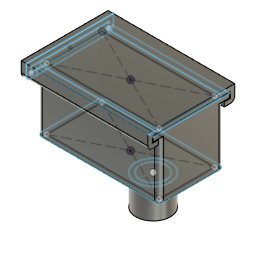
IRboxAugust v4 (Autodesk Fusion 360 design; units mm, degrees)
Autodesk Fusion 360 part; units mm, degrees
sketch "Sketch1" plane through (0, 0, 0) normal (0, 0, 1) x (1, 0, 0)
  line L0 (37.5, -18.5) -> (-37.5, -18.5)
  line L1 (-37.5, -18.5) -> (-37.5, 18.5)
  line L2 (-37.5, 18.5) -> (37.5, 18.5)
  line L3 (37.5, 18.5) -> (37.5, -18.5)
  line L4 (37.5, -18.5) -> (-37.5, 18.5) construction
  line L5 (-37.5, -18.5) -> (37.5, 18.5) construction
  line L6 (-37.5, 21.5) -> (37.5, 21.5)
  line L7 (40.5, 18.5) -> (40.5, -18.5)
  line L8 (37.5, -21.5) -> (-37.5, -21.5)
  line L9 (-40.5, -18.5) -> (-40.5, 18.5)
  arc A0 (-37.5, 21.5) -> (-40.5, 18.5) centre (-37.5, 18.5) ccw
  arc A1 (40.5, 18.5) -> (37.5, 21.5) centre (37.5, 18.5) ccw
  arc A2 (37.5, -21.5) -> (40.5, -18.5) centre (37.5, -18.5) ccw
  arc A3 (-40.5, -18.5) -> (-37.5, -21.5) centre (-37.5, -18.5) ccw
  circle A4 centre (20, -5) radius 8.5
  circle A5 centre (20, -5) radius 11.5
  dimension "d1" = 75
  dimension "d2" = 37
  dimension "d4" = 3
  dimension "d5" = 3
  dimension "d6" = 3
  dimension "d7" = 3
  dimension "d10" = 17
  dimension "d11" = 23
  constraint horizontal L0
  constraint perpendicular L0 L1
  constraint parallel L0 L2
  constraint parallel L1 L3
  constraint coincident L4 origin
  constraint coincident L5 origin
  constraint parallel L2 L6
  constraint parallel L3 L7
  constraint parallel L0 L8
  constraint parallel L1 L9
  constraint tangent L6 A0
  constraint tangent L9 A0
  constraint tangent L6 A1
  constraint tangent L7 A1
  constraint tangent L7 A2
  constraint tangent L8 A2
  constraint tangent L8 A3
  constraint tangent L9 A3
  constraint concentric A4 A5
  measures "d1" distance of L1.end L2.end
  measures "d2" distance of L0.end L1.end
  measures "d4" radius of A0
  measures "d5" radius of A1
  measures "d6" radius of A2
  measures "d7" radius of A3
  measures "d10" diameter of A4
  measures "d11" diameter of A5
extrude "Extrude2" add sketch "Sketch1" against normal blind 20 contours A5 makes body 1
extrude "Extrude1" add sketch "Sketch1" along normal blind 3 separate body contours L0 L1 L2 L3 | L6 L7 L8 L9 A0 A1 A2 A3 | A4 | A5 makes body 2
extrude "Extrude3" cut sketch "Sketch1" along normal blind 11 contours A4 bodies 2
extrude "Extrude4" add sketch "Sketch1" along normal blind 41 contours L6 L7 L8 L9 A0 A1 A2 A3 bodies 2
sketch "Sketch2" plane through (0, 0, 41) normal (0, 0, 1) x (-1, 0, 0)
  line L0 (37.5, -18.5) -> (-37.5, -18.5)
  line L1 (-37.5, -18.5) -> (-37.5, 18.5)
  line L2 (-37.5, 18.5) -> (37.5, 18.5)
  line L3 (37.5, 18.5) -> (37.5, -18.5)
  arc A0 (37.5, -21.5) -> (40.5, -18.5) centre (37.5, -18.5) ccw
  line L4 (40.5, -18.5) -> (40.5, 18.5)
  arc A1 (40.5, 18.5) -> (37.5, 21.5) centre (37.5, 18.5) ccw
  line L5 (37.5, 21.5) -> (-37.5, 21.5)
  arc A2 (-37.5, 21.5) -> (-40.5, 18.5) centre (-37.5, 18.5) ccw
  line L6 (-40.5, 18.5) -> (-40.5, -18.5)
  arc A3 (-40.5, -18.5) -> (-37.5, -21.5) centre (-37.5, -18.5) ccw
  line L7 (-37.5, -21.5) -> (37.5, -21.5)
  line L8 (37.5, -18.5) -> (-37.5, -18.5)
  line L9 (-37.5, -18.5) -> (-37.5, 18.5)
  line L10 (-37.5, 18.5) -> (37.5, 18.5)
  line L11 (37.5, 18.5) -> (37.5, -18.5)
  line L12 (37.5, -18.5) -> (-37.5, 18.5) construction
  line L13 (-37.5, -18.5) -> (37.5, 18.5) construction
  line L14 (37.5, -21.5) -> (-37.5, -21.5)
  line L15 (-40.5, -18.5) -> (-40.5, 18.5)
  line L16 (-37.5, 21.5) -> (37.5, 21.5)
  line L17 (40.5, 18.5) -> (40.5, -18.5)
  arc A4 (37.5, -21.5) -> (40.5, -18.5) centre (37.5, -18.5) ccw
  arc A5 (40.5, 18.5) -> (37.5, 21.5) centre (37.5, 18.5) ccw
  arc A6 (-40.5, -18.5) -> (-37.5, -21.5) centre (-37.5, -18.5) ccw
  arc A7 (-37.5, 21.5) -> (-40.5, 18.5) centre (-37.5, 18.5) ccw
  line L18 (37.5, -21.5) -> (-37.5, -21.5)
  line L19 (-37.5, -21.5) -> (-37.5, -25.5)
  line L20 (-37.5, -25.5) -> (37.5, -25.5)
  line L21 (37.5, -25.5) -> (37.5, -21.5)
  line L22 (37.5, 21.5) -> (-37.5, 21.5)
  line L23 (-37.5, 21.5) -> (-37.5, 25.5)
  line L24 (-37.5, 25.5) -> (37.5, 25.5)
  line L25 (37.5, 25.5) -> (37.5, 21.5)
  line L26 (-37.5, -25.5) -> (-40.5, -25.5)
  line L27 (-40.5, -25.5) -> (-40.5, 25.5)
  line L28 (-40.5, 25.5) -> (-37.5, 25.5)
  line L29 (-37.5, 25.5) -> (-37.5, -25.5)
  dimension "d19" = 3
  dimension "d20" = 3
  dimension "d21" = 3
  dimension "d22" = 3
  dimension "d23" = 4
  dimension "d24" = 4
  constraint horizontal L8
  constraint perpendicular L8 L9
  constraint parallel L8 L10
  constraint parallel L9 L11
  constraint coincident L0.start L3.end
  constraint coincident L12 origin
  constraint coincident L13 origin
  constraint parallel L8 L14
  constraint parallel L9 L15
  constraint parallel L10 L16
  constraint parallel L11 L17
  constraint tangent L14 A4
  constraint tangent L17 A4
  constraint tangent L16 A5
  constraint tangent L17 A5
  constraint tangent L14 A6
  constraint tangent L15 A6
  constraint tangent L15 A7
  constraint tangent L16 A7
  constraint horizontal L18
  constraint vertical L19
  constraint horizontal L20
  constraint vertical L21
  constraint horizontal L22
  constraint vertical L23
  constraint horizontal L24
  constraint vertical L25
  constraint horizontal L26
  constraint vertical L27
  constraint horizontal L28
  constraint vertical L29
  measures "d19" radius of A4
  measures "d20" radius of A5
  measures "d21" radius of A6
  measures "d22" radius of A7
  measures "d23" distance of A0.start L20.end
  measures "d24" distance of A1.end L24.end
extrude "Extrude6" add sketch "Sketch2" against normal blind 3 contours L1 A2 L6 A3 L9 L15 A6 A7 L27 L29 | A3 A6 L19 L26 L27 L29 | A2 A7 L23 L27 L28 L29 bodies 2
extrude "Extrude5" add sketch "Sketch2" against normal blind 3 contours L7 L14 L18 L19 L20 L21 L29 | L5 L16 L22 L23 L24 L25 L29 bodies 2
sketch "Sketch3" plane through (-40.5, 0, 0) normal (-1, 0, 0) x (0, -1, 0)
  line L0 (-18.5, 0) -> (18.5, 0)
  line L1 (18.5, 0) -> (18.5, 41)
  line L2 (18.5, 41) -> (-18.5, 41)
  line L3 (-18.5, 41) -> (-18.5, 0)
  line L4 (25.5, 38) -> (-25.5, 38)
  line L5 (-25.5, 38) -> (-25.5, 41)
  line L6 (-25.5, 41) -> (25.5, 41)
  line L7 (25.5, 41) -> (25.5, 38)
  line L8 (25.5, 38) -> (-25.5, 41) construction
  line L9 (-25.5, 38) -> (25.5, 41) construction
  line L10 (-26, 41.5) -> (26, 41.5)
  line L11 (26, 41.5) -> (26, 37.5)
  line L12 (26, 37.5) -> (-26, 37.5)
  line L13 (-26, 37.5) -> (-26, 41.5)
  line L14 (-29, 44.5) -> (29, 44.5)
  line L15 (29, 44.5) -> (29, 37.5)
  line L16 (26, 34.5) -> (-26, 34.5)
  line L17 (-29, 37.5) -> (-29, 44.5)
  line L18 (-22, 38) -> (-22, 34.5)
  line L19 (22, 38) -> (22, 34.5)
  arc A0 (-29, 37.5) -> (-26, 34.5) centre (-26, 37.5) ccw
  arc A1 (26, 34.5) -> (29, 37.5) centre (26, 37.5) ccw
  point P0 (0, 39.5)
  dimension "d29" = 51
  dimension "d30" = 3
  dimension "d31" = -0.5
  dimension "d33" = 3
  dimension "d34" = 3
  constraint horizontal L4
  constraint perpendicular L4 L5
  constraint parallel L4 L6
  constraint parallel L5 L7
  constraint coincident L8 P0
  constraint coincident L9 P0
  constraint coincident L4 L18.start
  constraint coincident L16 L18.end
  constraint perpendicular L16 L18
  constraint coincident L4 L19.start
  constraint coincident L16 L19.end
  constraint perpendicular L16 L19
  constraint parallel L6 L14
  constraint parallel L7 L15
  constraint parallel L4 L16
  constraint parallel L5 L17
  constraint tangent L16 A0
  constraint tangent L17 A0
  constraint tangent L15 A1
  constraint tangent L16 A1
  measures "d29" distance of L5.end L6.end
  measures "d30" distance of L4.end L5.end
  measures "d33" radius of A0
  measures "d34" radius of A1
extrude "Extrude7" add sketch "Sketch3" against normal blind 81 separate body contours L10 L11 L12 L13 L14 L15 L16 L17 L18 L19 A0 A1 makes body 3
extrude "Extrude8" add sketch "Sketch3" along normal blind 3.5 contours L10 L11 L12 L13 L14 L15 L16 L17 L18 L19 A0 A1 bodies 3
extrude "Extrude9" add sketch "Sketch3" along normal blind 3.5 contours L3 L12 L16 L18 | L1 L3 L12 L16 | L1 L12 L16 L19 | L3 L4 L12 L18 | L1 L3 L4 L12 | L10 L11 L12 L13 L14 L15 L16 L17 L18 L19 A0 A1 | L1 L4 L12 L19 | L3 L4 L5 L6 | L1 L2 L3 L4 L6 | L2 L4 L5 L6 L7 L10 L11 L12 L13 L18 L19 | L1 L4 L6 L7 bodies 3
extrude "Extrude10" cut sketch "Sketch3" along normal blind 0.5 contours L3 L12 L16 L18 | L1 L3 L12 L16 | L1 L12 L16 L19 | L3 L4 L12 L18 | L1 L3 L4 L12 | L1 L4 L12 L19 | L3 L4 L5 L6 | L1 L2 L3 L4 L6 | L2 L4 L5 L6 L7 L10 L11 L12 L13 L18 L19 | L1 L4 L6 L7 bodies 3
combine "Combine1" operation add target body 2 tool bodies 1
